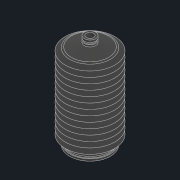
# Autodesk Inventor part: MCEN4000:T7
Saved by Autodesk Inventor 2021 (Build 250183000, 183)
## iProperties
Created: 2020-10-22
Part Number: MCEN4000:T7
Material: RUBBER, SILICONE
Document SubType Name: Modeling
Designer: Tang Kang Ning
Mass: 106.613 g
Surface Area: 1671.72 cm^2
Volume: 95.1898 cm^3
Density: 1.12 g/cm^3
Appearance: Rubber - Black
Description: BALL JOINT BELLOW
Author: Tang Kang Ning
Autodesk Inventor part; units mm, degrees
ref_plane "YZ Plane" through (0, 0, 0) normal (1, 0, 0) x (0, 1, 0)
ref_plane "XZ Plane" through (0, 0, 0) normal (0, 1, 0) x (-1, 0, 0)
ref_plane "XY Plane" through (0, 0, 0) normal (0, 0, 1) x (1, 0, 0)
sketch "Sketch2" plane through (0, 0, 0) normal (0, 0, 1) x (1, 0, 0)
  line L0 (37, 65.25) -> (-37, 65.25) projected
  line L1 (-9, 234.5) -> (9, 234.5) projected
  point P0 (0, 0)
  dimension "d47" = 169.25
  measures "d47" distance between parallel lines of L1 L0
sketch "Sketch1" plane through (0, 0, 0) normal (0, 0, 1) x (1, 0, 0)
  line L0 (-36.7449, 53.25) -> (37.2551, 53.25)
  line L1 (35, 65.25) -> (35, 53.25)
  line L2 (7.056, 234.5) -> (7.056, 222.5)
  line L3 (7.056, 234.5) -> (7.056, 222.5)
  line L4 (7.056, 234.5) -> (11.056, 234.5)
  line L5 (35, 53.25) -> (39, 53.25)
  line L6 (39, 53.25) -> (39, 57.25)
  line L7 (39, 57.25) -> (37, 57.25)
  line L8 (37, 57.25) -> (37, 61.25)
  line L9 (37, 61.25) -> (39, 61.25)
  line L10 (39, 61.25) -> (39, 65.25)
  line L11 (39, 65.25) -> (37, 65.25) construction
  line L12 (11.056, 234.5) -> (11.056, 230.5)
  line L13 (11.056, 230.5) -> (9.056, 230.5)
  line L14 (9.056, 230.5) -> (9.056, 226.5)
  line L15 (9.056, 226.5) -> (11.056, 226.5)
  line L16 (11.056, 226.5) -> (11.056, 223.0191)
  line L17 (39, 65.25) -> (47.4666, 70.5714)
  line L18 (37, 65.25) -> (45.4666, 70.5714)
  line L19 (37, 65.25) -> (37, 83.6946) construction
  line L20 (45.4666, 70.5714) -> (37, 70.5714) construction
  line L21 (45.4666, 70.5714) -> (37, 75.8928)
  line L22 (47.4666, 70.5714) -> (39, 75.8928)
  line L23 (37, 75.8928) -> (46.5513, 75.8928) construction
  line L24 (45.4666, 81.2141) -> (37, 86.5355)
  line L25 (47.4666, 81.2141) -> (39, 86.5355)
  line L26 (39, 75.8928) -> (47.4666, 81.2141)
  line L27 (37, 75.8928) -> (45.4666, 81.2141)
  line L28 (45.4666, 91.8569) -> (37, 97.1783)
  line L29 (47.4666, 91.8569) -> (39, 97.1783)
  line L30 (39, 86.5355) -> (47.4666, 91.8569)
  line L31 (37, 86.5355) -> (45.4666, 91.8569)
  line L32 (45.4666, 102.4996) -> (37, 107.821)
  line L33 (47.4666, 102.4996) -> (39, 107.821)
  line L34 (39, 97.1783) -> (47.4666, 102.4996)
  line L35 (37, 97.1783) -> (45.4666, 102.4996)
  line L36 (45.4666, 113.1424) -> (37, 118.4638)
  line L37 (47.4666, 113.1424) -> (39, 118.4638)
  line L38 (39, 107.821) -> (47.4666, 113.1424)
  line L39 (37, 107.821) -> (45.4666, 113.1424)
  line L40 (45.4666, 123.7851) -> (37, 129.1065)
  line L41 (47.4666, 123.7851) -> (39, 129.1065)
  line L42 (39, 118.4638) -> (47.4666, 123.7851)
  line L43 (37, 118.4638) -> (45.4666, 123.7851)
  line L44 (45.4666, 134.4279) -> (37, 139.7493)
  line L45 (47.4666, 134.4279) -> (39, 139.7493)
  line L46 (39, 129.1065) -> (47.4666, 134.4279)
  line L47 (37, 129.1065) -> (45.4666, 134.4279)
  line L48 (45.4666, 145.0706) -> (37, 150.392)
  line L49 (47.4666, 145.0706) -> (39, 150.392)
  line L50 (39, 139.7493) -> (47.4666, 145.0706)
  line L51 (37, 139.7493) -> (45.4666, 145.0706)
  line L52 (45.4666, 155.7134) -> (37, 161.0348)
  line L53 (47.4666, 155.7134) -> (39, 161.0348)
  line L54 (39, 150.392) -> (47.4666, 155.7134)
  line L55 (37, 150.392) -> (45.4666, 155.7134)
  line L56 (45.4666, 166.3561) -> (37, 171.6775)
  line L57 (47.4666, 166.3561) -> (39, 171.6775)
  line L58 (39, 161.0348) -> (47.4666, 166.3561)
  line L59 (37, 161.0348) -> (45.4666, 166.3561)
  line L60 (45.4666, 176.9989) -> (37, 182.3203)
  line L61 (47.4666, 176.9989) -> (39, 182.3203)
  line L62 (39, 171.6775) -> (47.4666, 176.9989)
  line L63 (37, 171.6775) -> (45.4666, 176.9989)
  line L64 (45.4666, 187.6417) -> (37, 192.963)
  line L65 (47.4666, 187.6417) -> (39, 192.963)
  line L66 (39, 182.3203) -> (47.4666, 187.6417)
  line L67 (37, 182.3203) -> (45.4666, 187.6417)
  line L68 (0, -37.6229) -> (0, 264.2373)
  line L69 (9.056, 222.5) -> (7.056, 222.5)
  line L70 (37, 65.25) -> (35, 65.25)
  line L71 (0, 208431.7305) -> (0, -209414.2305)
  line L72 (37, 65.25) -> (-37, 65.25) projected
  line L73 (37, 65.25) -> (-37, 65.25) construction
  line L74 (37, 65.25) -> (35, 65.25)
  line L75 (7.056, 222.5) -> (9.056, 222.5)
  line L76 (11.056, 223.0191) -> (7.056, 224.2003)
  line L77 (45.4666, 198.2844) -> (37, 203.6058)
  line L78 (47.4666, 198.2844) -> (39, 203.6058)
  line L79 (39, 192.963) -> (47.4666, 198.2844)
  line L80 (37, 192.963) -> (45.4666, 198.2844)
  line L81 (45.4666, 208.9272) -> (37, 214.2485)
  line L82 (47.4666, 208.9272) -> (39, 214.2485)
  line L83 (39, 203.6058) -> (47.4666, 208.9272)
  line L84 (37, 203.6058) -> (45.4666, 208.9272)
  line L85 (9.056, 222.5) -> (37, 214.2485)
  line L86 (7.056, 224.2003) -> (35.6774, 215.7488)
  arc A0 (39, 214.2485) -> (35.6774, 215.7488) centre (31.8976, 202.9482) ccw
  point P0 (0, 0)
  point P1 (39, 75.8928)
  point P2 (39, 86.5355)
  point P3 (39, 97.1783)
  point P4 (39, 107.821)
  point P5 (39, 118.4638)
  point P6 (39, 129.1065)
  point P7 (39, 139.7493)
  point P8 (39, 150.392)
  point P9 (39, 161.0348)
  point P10 (39, 171.6775)
  point P11 (39, 182.3203)
  point P12 (7, 203.6144)
  point P13 (39, 192.963)
  point P14 (9, 223.6095)
  point P15 (9, 222.5)
  point P16 (11.056, 223.0191)
  dimension "d0" = 4
  dimension "d1" = 12
  dimension "d2" = 4
  dimension "d3" = 2
  dimension "d4" = 2
  dimension "d5" = 4
  dimension "d7" = 2
  dimension "d8" = 2
  dimension "d12" = 122.15
  dimension "d13" = 1.0643
  dimension "d17" = 10
  dimension "d18" = 10.6427
  dimension "d28" = 10.6427
  dimension "d34" = 12
  dimension "d37" = 7.056
  dimension "d39" = 169.25
  dimension "d46" = 2
  dimension "d48" = 1.0643
  dimension "d49" = 4
  constraints: 170 end point, 13 perpendicular, 9 point on line, 5 vertical, 3 collinear, 3 horizontal, 3 parallel, 2 point on circle, 2 tangent, 1 centre point, 1 coincident, 1 equal length, 134 other
  measures "d0" distance between parallel lines of L11 L9
  measures "d1" distance of L1.start L1.end
  measures "d2" distance between parallel lines of L5 L7
  measures "d3" distance between parallel lines of L8 L10
  measures "d4" distance between parallel lines of L1 L8
  measures "d5" distance of L4.end L12.end
  measures "d7" distance between parallel lines of L2 L14
  measures "d8" distance between parallel lines of L14 L16
  measures "d12" angle of L10 L17
  measures "d13" distance between parallel lines of L17 L18
  measures "d17" distance of L10.end L17.end
  measures "d18" distance of L11.end L21.end
  measures "d28" distance of L18.end L24.start
  measures "d34" distance of L2.end L2.start
  measures "d37" distance between parallel lines of L2 L68
  measures "d39" distance between parallel lines of L69 L0
  measures "d46" distance of L2.end L69.start
  measures "d48" distance between parallel lines of L85 L76
  measures "d49" distance between parallel lines of L13 L15
revolve "Revolution1" add sketch "Sketch1" angle 360 about axis through (0, -37.6229, 0) along (0, 1, 0) contours L1 L70 L18 L21 L27 L24 L31 L28 L35 L32 L39 L36 L43 L40 L47 L44 L51 L48 L55 L52 L59 L56 L63 L60 L67 L64 L80 L77 L84 L81 L85 L69 L2 L76 L86 A0 L82 L83 L78 L79 L65 L66 L61 L62 L57 L58 L53 L54 L49 L50 L45 L46 L41 L42 L37 L38 L33 L34 L29 L30 L25 L26 L22 L17 L10 L9 L8 L7 L6 L5 L0 | L2 L4 L12 L13 L14 L15 L16 L76
equation "\"d0\" = 0.333333 * d1"
equation "\"d2\" = d0"
equation "\"d5\" = d0"
equation "\"d37\" = RevolveDIA"
equation "\"d10\" = d9"
equation "\"RevolveDIA\" = 7.055999"
equation "\"d9\" = 171.191599"
body "Solid1"
